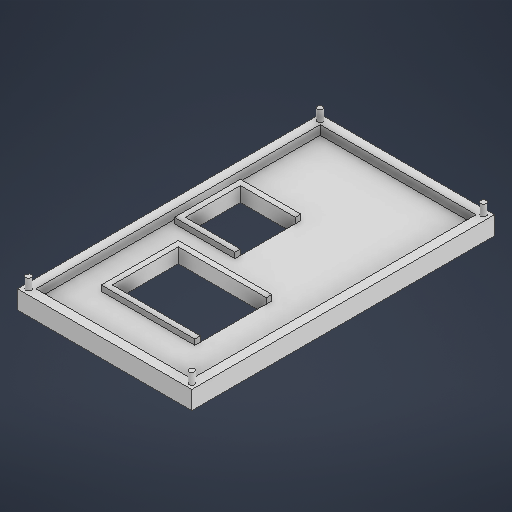
# Autodesk Inventor part: 零件3
Saved by Autodesk Inventor 2026.2 (Build 302298000, 298)
## iProperties
Created: 2025-12-21
Part Number: 零件3
Material: 一般
Document SubType Name: Modeling
Designer: USER
Density: 1 g/cm^3
Appearance: 預設
Author: USER
Autodesk Inventor part; units mm, degrees
ref_plane "YZ Plane" through (0, 0, 0) normal (1, 0, 0) x (0, 1, 0)
ref_plane "XZ Plane" through (0, 0, 0) normal (0, 1, 0) x (-1, 0, 0)
ref_plane "XY Plane" through (0, 0, 0) normal (0, 0, 1) x (1, 0, 0)
sketch "草圖1" plane through (0, 0, 0) normal (0, 1, 0) x (-1, 0, 0)
  line L0 (0, 0) -> (95, 0)
  line L1 (95, 0) -> (95, -165)
  line L2 (95, -165) -> (0, -165)
  line L3 (0, -165) -> (0, 0)
  dimension "d0" = 95
  dimension "d1" = 165
  constraints: 8 end point, 2 parallel, 1 horizontal, 1 perpendicular
  measures "d0" distance of L1.end L2.end
  measures "d1" distance of L0.end L1.end
extrude "擠出1" add sketch "草圖1" along normal blind 5
sketch "草圖2" plane through (0, 5, 0) normal (0, 1, 0) x (1, 0, 0)
  circle A0 centre (-3, 3) radius 1.5
  line L0 (0, 0) -> (0, 165) projected
  line L1 (-95, 0) -> (0, 0) projected
  circle A1 centre (-92, 3) radius 1.5
  line L2 (-95, 165) -> (-95, 0) projected
  circle A2 centre (-92, 162) radius 1.5
  line L3 (0, 165) -> (-95, 165) projected
  circle A3 centre (-3, 162) radius 1.5
  dimension "d4" = 3
  dimension "d5" = 3
  dimension "d6" = 3
  dimension "d7" = 3
  dimension "d8" = 3
  dimension "d9" = 3
  dimension "d10" = 3
  dimension "d11" = 3
  dimension "d12" = 3
  dimension "d13" = 3
  dimension "d14" = 3
  dimension "d15" = 3
  constraints: 4 centre point
  measures "d4" diameter of A0
  measures "d5" distance from line of L0 A0.centre
  measures "d6" distance from line of L1 A0.centre
  measures "d7" diameter of A1
  measures "d8" distance from line of L2 A1.centre
  measures "d9" distance from line of L1 A1.centre
  measures "d10" diameter of A2
  measures "d11" distance from line of L3 A2.centre
  measures "d12" distance from line of L2 A2.centre
  measures "d13" diameter of A3
  measures "d14" distance from line of L3 A3.centre
  measures "d15" distance from line of L0 A3.centre
extrude "擠出2" add sketch "草圖2" along normal blind 11 contours A0 | A1 | A2 | A3
sketch "草圖3" plane through (0, 0, 0) normal (0, -1, 0) x (1, 0, 0)
  line L0 (-25, -60.15) -> (-20, -60.15)
  line L1 (-20, -60.15) -> (-20, -35.15)
  line L2 (-20, -35.15) -> (-25, -35.15)
  line L3 (-25, -35.15) -> (-25, -60.15)
  line L4 (-95, 0) -> (0, 0) projected
  line L5 (0, 0) -> (0, -165) projected
  line L6 (-73, -65.65) -> (-25, -65.65)
  line L7 (-25, -65.65) -> (-25, -29.65)
  line L8 (-25, -29.65) -> (-73, -29.65)
  line L9 (-73, -29.65) -> (-73, -65.65)
  point P0 (-22.5, -35.15)
  point P1 (-20, -47.65)
  point P2 (-25, -47.65)
  dimension "d18" = 35.15
  dimension "d19" = 20
  dimension "d20" = 5
  dimension "d21" = 25
  dimension "d22" = 48
  dimension "d23" = 36
  dimension "d24" = 0
  dimension "d25" = 29.65
  constraints: 16 end point, 4 parallel, 3 midpoint, 2 horizontal, 2 perpendicular
  measures "d18" distance from line of L4 point (-22.5, -35.15)
  measures "d19" distance from line of L5 point (-20, -47.65)
  measures "d20" distance of L1.end L2.end
  measures "d21" distance of L2.end L0.start
  measures "d22" distance of L6.start L6.end
  measures "d23" distance of L6.end L7.end
  measures "d24" distance from line of L3 point (-25, -47.65)
  measures "d25" distance between parallel lines of L4 L8
extrude "擠出3" cut sketch "草圖3" against normal blind 6 contours L7 L6 L9 L8 L3
sketch "草圖4" plane through (0, 0, 0) normal (0, -1, 0) x (1, 0, 0)
  line L0 (-85, -81.5) -> (-55, -81.5)
  line L1 (-55, -81.5) -> (-55, -111.5)
  line L2 (-55, -111.5) -> (-85, -111.5)
  line L3 (-85, -111.5) -> (-85, -81.5)
  line L4 (0, -165) -> (-95, -165) projected
  line L5 (-95, -165) -> (-95, 0) projected
  point P0 (0, 0)
  point P1 (-85, -96.5)
  dimension "d28" = 30
  dimension "d29" = 30
  dimension "d30" = 83.5
  dimension "d31" = 10
  constraints: 8 end point, 2 parallel, 1 horizontal, 1 midpoint, 1 perpendicular
  measures "d28" distance of L0.start L0.end
  measures "d29" distance of L2.end L0.start
  measures "d30" distance between parallel lines of L0 L4
  measures "d31" distance from line of point (-85, -96.5) L5
extrude "擠出4" cut sketch "草圖4" against normal blind 6
sketch "草圖5" plane through (0, 5, 0) normal (0, 1, 0) x (1, 0, 0)
  line L0 (-25, 26.65) -> (-76, 26.65)
  line L1 (-76, 26.65) -> (-76, 68.65)
  line L2 (-76, 68.65) -> (-25, 68.65)
  line L3 (-25, 68.65) -> (-25, 26.65)
  line L4 (-25, 29.65) -> (-73, 29.65) projected
  line L5 (-25, 65.65) -> (-25, 29.65) projected
  line L6 (-73, 65.65) -> (-25, 65.65) projected
  line L7 (-73, 29.65) -> (-73, 65.65) projected
  point P0 (0, 0)
  point P1 (-70, 65.65)
  point P2 (-70, 29.65)
  dimension "d34" = 3
  dimension "d35" = 0
  dimension "d36" = 3
  dimension "d40" = 3
  constraints: 8 end point, 2 parallel, 1 horizontal, 1 perpendicular
  measures "d34" distance between parallel lines of L0 L4
  measures "d35" distance between parallel lines of L3 L5
  measures "d36" distance between parallel lines of L6 L2
  measures "d40" distance between parallel lines of L1 L7
extrude "擠出5" add sketch "草圖5" along normal blind 3 contours L0 L1 L2 L3 L6 L7 L4
sketch "草圖6" plane through (0, 5, 0) normal (0, 1, 0) x (1, 0, 0)
  line L0 (-88, 78.5) -> (-55, 78.5)
  line L1 (-55, 78.5) -> (-55, 114.5)
  line L2 (-55, 114.5) -> (-88, 114.5)
  line L3 (-88, 114.5) -> (-88, 78.5)
  line L4 (-85, 81.5) -> (-85, 111.5) projected
  line L5 (-55, 81.5) -> (-85, 81.5) projected
  line L6 (-85, 111.5) -> (-55, 111.5) projected
  line L7 (-55, 111.5) -> (-55, 81.5) projected
  point P0 (0, 0)
  dimension "d41" = 3
  dimension "d42" = 3
  dimension "d43" = 3
  dimension "d44" = 0
  constraints: 8 end point, 2 parallel, 1 horizontal, 1 perpendicular
  measures "d41" distance between parallel lines of L3 L4
  measures "d42" distance between parallel lines of L0 L5
  measures "d43" distance between parallel lines of L2 L6
  measures "d44" distance between parallel lines of L7 L1
extrude "擠出6" add sketch "草圖6" along normal blind 3 contours L3 L2 L1 L6 L4 L5 L0
sketch "草圖7" plane through (0, 5, 0) normal (0, 1, 0) x (1, 0, 0)
  line L0 (-95, 0) -> (0, 0)
  line L1 (0, 0) -> (0, 165)
  line L2 (0, 165) -> (-95, 165)
  line L3 (-95, 165) -> (-95, 0)
  line L4 (-95, 165) -> (-95, 0) projected
  line L5 (0, 165) -> (-95, 165) projected
  line L6 (0, 0) -> (0, 165) projected
  line L7 (-95, 0) -> (0, 0) projected
  line L8 (-90, 5) -> (-5, 5)
  line L9 (-5, 5) -> (-5, 160)
  line L10 (-5, 160) -> (-90, 160)
  line L11 (-90, 160) -> (-90, 5)
  dimension "d47" = 5
  dimension "d48" = 5
  dimension "d49" = 5
  dimension "d50" = 5
  constraints: 16 end point, 4 collinear, 4 parallel, 2 horizontal, 2 perpendicular
  measures "d47" distance between parallel lines of L3 L11
  measures "d48" distance between parallel lines of L2 L10
  measures "d49" distance between parallel lines of L0 L8
  measures "d50" distance between parallel lines of L1 L9
extrude "擠出7" add sketch "草圖7" along normal blind 5
